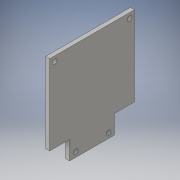
# Autodesk Inventor part: pixy
Saved by Autodesk Inventor 2016 (Build 200138000, 138)
## iProperties
Created: 2015-09-30
Part Number: pixy
Material: Generic
Document SubType Name: Modeling
Designer: Hulbert Office
Density: 1 g/cm^3
Appearance: Default
Author: Hulbert Office
Autodesk Inventor part; units mm, degrees
ref_plane "YZ Plane" through (0, 0, 0) normal (1, 0, 0) x (0, 1, 0)
ref_plane "XZ Plane" through (0, 0, 0) normal (0, 1, 0) x (-1, 0, 0)
ref_plane "XY Plane" through (0, 0, 0) normal (0, 0, 1) x (1, 0, 0)
sketch "Sketch1" plane through (0, 0, 0) normal (1, 0, 0) x (0, 1, 0)
  line L0 (35.3248, 26.5797) -> (35.3248, -27.2683)
  line L1 (35.3248, -27.2683) -> (-15.4752, -27.2683)
  line L2 (-15.4752, -27.2683) -> (-15.4752, -14.5683)
  line L3 (-15.4752, -14.5683) -> (-27.319, -14.5683)
  line L4 (-27.319, -14.5683) -> (-27.319, 13.8797)
  line L5 (-27.319, 13.8797) -> (-15.4752, 13.8797)
  line L6 (-15.4752, 13.8797) -> (-15.4752, 26.5797)
  line L7 (-15.4752, 26.5797) -> (35.3248, 26.5797)
  line L8 (-27.319, -0.3443) -> (-33.7293, -0.3443)
  circle A0 centre (32.1498, 23.4047) radius 1.524
  circle A1 centre (32.1498, -24.0933) radius 1.524
  circle A2 centre (-24.144, -10.7583) radius 1.524
  circle A3 centre (-24.144, 10.0697) radius 1.524
  point P0 (0, 0)
  dimension "d0" = 53.848
  dimension "d1" = 12.7
  dimension "d2" = 12.7
  dimension "d3" = 26.924
  dimension "d4" = 50.8
  dimension "d5" = 3.048
  dimension "d6" = 3.048
  dimension "d7" = 3.048
  dimension "d8" = 3.048
  dimension "d9" = 3.175
  dimension "d10" = 3.175
  dimension "d11" = 3.175
  dimension "d12" = 3.175
  dimension "d13" = 16.51
  dimension "d14" = 16.51
  dimension "d15" = 3.175
  dimension "d16" = 3.175
  constraints: 18 end point, 5 perpendicular, 4 centre point, 2 point on line, 1 horizontal, 1 midpoint, 1 vertical
  measures "d0" distance of L0.start L0.end
  measures "d1" distance of L5.end L6.end
  measures "d2" distance of L1.end L2.end
  measures "d3" vertical distance of L1.end L8.start
  measures "d4" distance of L6.end L0.start
  measures "d5" diameter of A0
  measures "d6" diameter of A1
  measures "d7" diameter of A2
  measures "d8" diameter of A3
  measures "d9" distance from line of L0 A0.centre
  measures "d10" distance from line of L7 A0.centre
  measures "d11" distance from line of L1 A1.centre
  measures "d12" distance from line of L0 A1.centre
  measures "d13" vertical distance of L1.end A2.centre
  measures "d14" distance from line of L7 A3.centre
  measures "d15" distance from line of L4 A2.centre
  measures "d16" distance from line of L4 A3.centre
extrude "Extrusion1" add sketch "Sketch1" along normal blind 2.54
body "Solid1"
